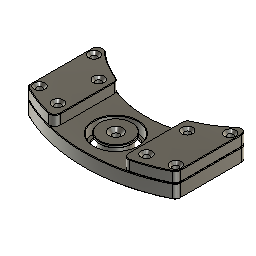
Router Hole Jig v2 (Autodesk Fusion 360 design; units mm, degrees)
Autodesk Fusion 360 part; units mm, degrees
sketch "Sketch1" plane through (0, 0, 0) normal (0, 0, 1) x (1, 0, 0)
  circle A0 centre (0, 0) radius 72.5 construction
  line L0 (-55, 47.2361) -> (-55, -47.2361) construction
  line L1 (55, 47.2361) -> (55, -47.2361) construction
  circle A1 centre (0, -95) radius 16
  line L2 (-55, -47.8478) -> (-55, -105)
  line L3 (55, -47.8478) -> (55, -105)
  arc A2 (-55, -47.8478) -> (55, -47.8478) centre (0, 0) ccw
  arc A3 (-55, -105) -> (55, -105) centre (0, 0) ccw
  circle A4 centre (0, -95) radius 14
  line L4 (-32.5, -75) -> (32.5, -75) construction
  line L5 (32.5, -75) -> (32.5, -105) construction
  line L6 (32.5, -105) -> (-32.5, -105) construction
  line L7 (-32.5, -105) -> (-32.5, -75) construction
  line L8 (-32.5, -75) -> (32.5, -105) construction
  line L9 (32.5, -75) -> (-32.5, -105) construction
  line L10 (-50, -61) -> (50, -61) construction
  line L11 (50, -61) -> (50, -101) construction
  line L12 (50, -101) -> (-50, -101) construction
  line L13 (-50, -101) -> (-50, -61) construction
  line L14 (-50, -61) -> (50, -101) construction
  line L15 (50, -61) -> (-50, -101) construction
  circle A5 centre (-50, -101) radius 2.9
  circle A6 centre (-50, -61) radius 2.9
  circle A7 centre (-32.5, -75) radius 2.9
  circle A8 centre (-32.5, -105) radius 2.9
  circle A9 centre (32.5, -105) radius 2.9
  circle A10 centre (32.5, -75) radius 2.9
  circle A11 centre (50, -61) radius 2.9
  circle A12 centre (50, -101) radius 2.9
  line L16 (-25, -68.4793) -> (-25, -115.8663)
  line L17 (25, -115.8663) -> (25, -68.4793)
  circle A13 centre (0, -95) radius 10
  circle A14 centre (0, -95) radius 12
  point P0 (0, -90)
  point P1 (0, -81)
  dimension "d1" = 145
  dimension "d2" = 110
  dimension "d3" = 32
  dimension "d4" = 0.4
  dimension "d5" = 95
  dimension "d7" = 105
  dimension "d14" = 28
  dimension "d20" = 30
  dimension "d21" = 65
  dimension "d22" = 5
  dimension "d25" = 100
  dimension "d26" = 40
  dimension "d27" = 14
  dimension "d28" = 5.8
  dimension "d32" = 30
  dimension "d45" = 20
  dimension "d46" = 24
  constraint coincident A0.centre A2.centre
  constraint coincident A0 L0.start
  constraint coincident A0 L0.end
  constraint vertical L0
  constraint coincident A0 L1.start
  constraint coincident A0 L1.end
  constraint parallel L0 L1
  constraint horizontal L0.start L1.start
  constraint parallel L0 L2
  constraint vertical L3
  constraint coincident L3.start A2.end
  constraint collinear L1 L3
  constraint collinear L0 L2
  constraint vertical A1.centre A0.centre
  constraint concentric A1 A4
  constraint horizontal L4
  constraint perpendicular L4 L5
  constraint parallel L4 L6
  constraint parallel L5 L7
  constraint coincident L8 P0
  constraint coincident L9 P0
  constraint vertical A0.centre P0
  constraint horizontal L10
  constraint perpendicular L10 L11
  constraint parallel L10 L12
  constraint parallel L11 L13
  constraint coincident L14 P1
  constraint coincident L15 P1
  constraint vertical A0.centre P1
  constraint coincident L12.end L13.start
  constraint coincident L10.start L13.end
  constraint coincident L4.start L7.end
  constraint coincident L6.end L7.start
  constraint coincident L5.end L6.start
  constraint coincident L4.end L5.start
  constraint coincident L10.end L11.start
  constraint coincident L11.end L12.start
  constraint equal A11 A12
  constraint equal A10 A11
  constraint equal A9 A10
  constraint equal A8 A9
  constraint equal A7 A8
  constraint equal A6 A7
  constraint equal A5 A6
  constraint coincident A2 L16.start
  constraint coincident A3 L16.end
  constraint perpendicular L6 L16
  constraint coincident A3 L17.start
  constraint coincident A2 L17.end
  constraint parallel L16 L17
  constraint horizontal L16.end L17.start
  constraint concentric A4 A13
  constraint concentric A1 A14
  measures "d1" diameter of A0
  measures "d2" distance of L0 L1
  measures "d3" diameter of A1
  measures "d4" distance of A0 A2
  measures "d5" distance of A0.centre A1.centre
  measures "d7" vertical distance of L3.end A0.centre
  measures "d14" diameter of A4
  measures "d20" distance of L4.end L5.end
  measures "d21" distance of L5.end L6.end
  measures "d22" distance of A1.centre P0
  measures "d25" distance of L10.start L10.end
  measures "d26" distance of L10.start L12.end
  measures "d27" distance of A1.centre P1
  measures "d28" diameter of A6
  measures "d32" distance of L2 L16
  measures "d45" diameter of A13
  measures "d46" diameter of A14
sketch "Sketch2" plane through (0, 0, 0) normal (0, 1, 0) x (1, 0, 0)
  line L0 (-55, 0) -> (55, 0)
  line L1 (55, 0) -> (55, -18)
  line L2 (55, -18) -> (-55, -18)
  line L3 (-55, -18) -> (-55, 0)
  line L4 (-42, -10) -> (42, -10) construction
  line L5 (0, -10) -> (0, 0) construction
  circle A0 centre (42, -10) radius 4
  circle A1 centre (-42, -10) radius 4
  line L6 (-55, -10) -> (-46, -10)
  line L7 (46, -10) -> (55, -10)
  line L8 (-38, -10) -> (38, -10)
  line L9 (-46, -10) -> (-38, -10)
  line L10 (38, -10) -> (46, -10)
  point P0 (-55, 0)
  point P1 (55, 0)
  dimension "d8" = 18
  dimension "d9" = 84
  dimension "d10" = 8
  dimension "d11" = 10
  dimension "d12" = 10
  dimension "d13" = 10
  constraint horizontal L0
  constraint vertical L1
  constraint horizontal L2
  constraint vertical L3
  constraint coincident P0 L0.start
  constraint coincident P1 L0.end
  constraint parallel L2 L4
  constraint midpoint L4 L5.start
  constraint coincident L5.end origin
  constraint vertical L5
  constraint equal A0 A1
  constraint coincident L3 L6.start
  constraint coincident A1 L6.end
  constraint perpendicular L3 L6
  constraint coincident A0 L7.start
  constraint coincident L1 L7.end
  constraint perpendicular L1 L7
  constraint collinear L6 L7
  constraint coincident A1 L8.start
  constraint coincident A0 L8.end
  constraint parallel L6 L8
  constraint coincident L4.end A0.centre
  constraint coincident L4.start A1.centre
  measures "d8" distance of P1 L1.end
  measures "d9" distance of L4.start L4.end
  measures "d10" diameter of A1
  measures "d11" distance of L5.start L5.end
  measures "d12" distance of P0 L6
  measures "d13" distance of L0 L8
extrude "Extrude1" add sketch "Sketch1" along normal blind 2 contours A1 | L2 A2 A3 L16 | A2 A3 L16 L17 | L3 A2 A3 L17 | A5 | A6 | A7 | A8 | A9 | A10 | A11 | A12 makes body 1
extrude "Extrude2" add sketch "Sketch1" along normal blind 18 contours L2 A2 A3 L16 | A2 A3 L16 L17 | L3 A2 A3 L17 | A5 | A6 | A7 | A8 | A9 | A10 | A11 | A12 bodies 1
extrude "Extrude3" cut sketch "Sketch2" against normal through all contours L1 L2 L3 A0 A1 L6 L7 L8 | A1 L9 | A0 L10 picked at (-43.2741, -12.2068) picked at (43.146, -11.3428) bodies 1
extrude "Extrude4" cut sketch "Sketch2" against normal blind 105 contours A1 L9 | A1 L9 | A0 L10 | A0 L10 bodies 1
extrude "Extrude5" cut sketch "Sketch1" against normal blind 8.5 from surface at 10 contours A5 | A6 | A7 | A8 | A9 | A10 | A11 | A12 bodies 1
extrude "Extrude6" add sketch "Sketch1" against normal blind 7.8 from surface at 18 separate body contours L2 A2 A3 L16 | L3 A2 A3 L17 | A5 | A6 | A7 | A8 | A9 | A10 | A11 | A12 makes body 2 at (-35.2176, -97.0493, 18) makes body 3 at (35.2176, -97.0493, 18)
extrude "Extrude7" cut sketch "Sketch2" against normal blind 105 contours A1 L9 | A1 L9 | A0 L10 | A0 L10 bodies 2 3
sketch "Sketch3" plane through (0, 0, 18) normal (0, 0, 1) x (-1, 0, 0)
  arc A0 (-25, 115.8663) -> (-55, 105) centre (0, 0) ccw
  line L0 (-55, 105) -> (-55, 47.8478)
  arc A1 (-25, 68.4793) -> (-55, 47.8478) centre (0, 0) ccw
  line L1 (-25, 68.4793) -> (-25, 115.8663)
  point P0 (-32.5, 75)
  point P1 (-50, 61)
  point P2 (-50, 101)
  point P3 (-32.5, 105)
  point P4 (32.5, 105)
  point P5 (32.5, 75)
  point P6 (50, 61)
  point P7 (50, 101)
hole "Hole1" at (-50, -101, 18) at (-50, -61, 18) at (-32.5, -75, 18) at (-32.5, -105, 18) at (32.5, -75, 18) at (32.5, -105, 18) at (50, -101, 18) at (50, -61, 18) direction (0, 0, -1) diameter 4.4 depth 12 tip angle 118 countersink diameter 8 countersink angle 90 bodies 2 3
fillet "Fillet1" radius 4 12 edges at (-55, -47.8478, 5) (55, -47.8478, 5) (-55, -105, 5) (55, -105, 5) (-55, -47.8478, 14.1) (-25, -68.4793, 14.1) (-55, -105, 14.1) (-25, -115.8663, 14.1) (25, -68.4793, 14.1) (55, -47.8478, 14.1) (25, -115.8663, 14.1) (55, -105, 14.1) on bodies 1 2 3
extrude "Extrude8" add sketch "Sketch1" along normal blind 9 and the other way blind 0.2 separate body contours A13 makes body 4
extrude "Extrude9" add sketch "Sketch1" along normal blind 2 from surface at 9 contours A13 | A14 bodies 4
hole "Hole2" at (0, -95, 11) direction (0, 0, -1) diameter 5 depth 12 tip angle 118 countersink diameter 10 countersink angle 90 bodies 4
chamfer "Chamfer1" distance 0.4 angle 45 59 edges at (-11.1879, -99.3394, 11) (-11.1879, -90.6606, 9) (-9.3233, -98.6162, 9) (-9.3233, -91.3838, -0.2) (-2.3308, -95.904, -0.2) (38.4687, -61.9239, 18) (52.6415, -53.9076, 18) (55, -80.0532, 18) (54.4003, -104.6577, 18) (41.6165, -110.9868, 18) (26.5557, -113.9668, 18) (25, -91.0114, 18) (25.6808, -68.99, 18) (32.8556, -65.0762, 10.2) (47.1817, -55.5725, 10.2) (52.6415, -53.9076, 10.2) (55, -80.0532, 10.2) (54.4003, -104.6577, 10.2) (41.6165, -110.9868, 10.2) (26.5557, -113.9668, 10.2) (25, -91.0114, 10.2) (25.6808, -68.99, 10.2) (-41.6165, -110.9868, 10.2) (-54.4003, -104.6577, 10.2) (-55, -80.0532, 10.2) (-52.6415, -53.9076, 10.2) (-47.1817, -55.5725, 10.2) (-32.8556, -65.0762, 10.2) (-25.6808, -68.99, 10.2) (-25, -91.0114, 10.2) (-26.5557, -113.9668, 10.2) (-55, -80.0532, 18) (-54.4003, -104.6577, 18) (-41.6165, -110.9868, 18) (-26.5557, -113.9668, 18) (-25, -91.0114, 18) (-25.6808, -68.99, 18) (-38.4687, -61.9239, 18) (-52.6415, -53.9076, 18) (0, -118.5327, 0) (54.4003, -104.6577, 0) (55, -80.0532, 0) (52.6415, -53.9076, 0) (0, -72.9, 0) (-52.6415, -53.9076, 0) (-55, -80.0532, 0) (-54.4003, -104.6577, 0) (-13.0526, -89.9374, 0) (-14.9172, -100.7858, 10) (0, -118.5327, 10) (-54.4003, -104.6577, 10) (-55, -80.0532, 10) (-52.6415, -53.9076, 10) (-47.1841, -55.5704, 10) (47.1841, -55.5704, 10) (52.6415, -53.9076, 10) (55, -80.0532, 10) (54.4003, -104.6577, 10) (0, -72.9, 10) on bodies 1 2 3 4
